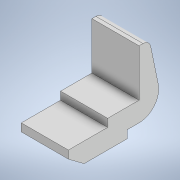
# Autodesk Inventor part: HangerJaw
Saved by Autodesk Inventor 2022.2 (Build 262287030, 287C)
## iProperties
Created: 2023-03-17
Part Number: HangerJaw
Material: Generic
Document SubType Name: Modeling
Designer: jak27277
Density: 1 g/cm^3
Appearance: Default
Author: jak27277
Autodesk Inventor part; units mm, degrees
ref_plane "YZ Plane" through (0, 0, 0) normal (1, 0, 0) x (0, 1, 0)
ref_plane "XZ Plane" through (0, 0, 0) normal (0, 1, 0) x (-1, 0, 0)
ref_plane "XY Plane" through (0, 0, 0) normal (0, 0, 1) x (1, 0, 0)
sketch "Sketch1" plane through (0, 0, 0) normal (1, 0, 0) x (0, 1, 0)
  line L0 (76.2, 0) -> (0, 0)
  line L1 (0, 0) -> (0, 50.8)
  line L2 (0, 50.8) -> (-12.7, 50.8)
  line L3 (-12.7, 50.8) -> (-12.7, 114.3)
  line L4 (-12.7, 114.3) -> (-25.4, 114.3)
  line L5 (-25.4, 114.3) -> (-44.45, 88.9)
  line L6 (-44.45, 88.9) -> (-44.45, 19.05)
  line L7 (-44.45, 19.05) -> (-31.75, 19.05)
  line L8 (-31.75, 19.05) -> (-31.75, 0)
  arc A0 (-31.75, 0) -> (6.4155, -31.0951) centre (0, 0) ccw
  line L9 (6.4155, -31.0951) -> (66.0662, -18.788)
  arc A1 (66.0662, -18.788) -> (76.2, -6.35) centre (63.5, -6.35) ccw
  line L10 (76.2, -6.35) -> (76.2, 0)
  dimension "d0" = 120.65
  dimension "d1" = 69.85
  dimension "d2" = 31.75
  dimension "d3" = 31.75
  dimension "d4" = 12.7
  dimension "d5" = 6.35
  dimension "d6" = 76.2
  dimension "d7" = 12.7
  dimension "d8" = 12.7
  dimension "d9" = 114.3
  dimension "d10" = 50.8
  dimension "d11" = 19.05
  dimension "d12" = 0
  constraints: 22 end point, 7 perpendicular, 4 point on circle, 4 tangent, 2 centre point, 1 horizontal, 1 parallel
  measures "d0" distance between parallel lines of L6 L10
  measures "d1" distance of L5.end L6.end
  measures "d2" distance between parallel lines of L1 L8
  measures "d3" radius of A0
  measures "d4" radius of A1
  measures "d5" distance of L10.start L0.start
  measures "d6" distance of L0.start L0.end
  measures "d7" distance of L1.end L2.end
  measures "d8" distance of L3.end L4.end
  measures "d9" distance between parallel lines of L4 L0
  measures "d10" distance of L0.end L1.end
  measures "d11" distance of L7.end L8.end
  measures "d12" distance of L0.end A0.centre
extrude "Extrusion1" add sketch "Sketch1" along normal blind 76.2
body "Solid1"
